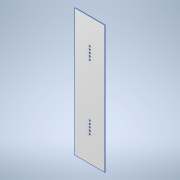
# Autodesk Inventor part: 7001_Aluminum_Chasis_Coil_Assembly_Separator_Tx_Filter_MPSv2_v1
Saved by Autodesk Inventor 2021 (Build 250183000, 183)
## iProperties
Created: 2020-11-18
Part Number: 7001_Aluminum_Chasis_Coil_Assembly_Separator_Tx_Filter_MPSv2_v1
Material: Aluminum 6061
Document SubType Name: Modeling
Designer: Admin
Density: 2.7 g/cm^3
Appearance: Aluminum - Flat
Author: Admin
Autodesk Inventor part; units mm, degrees
ref_plane "YZ Plane" through (0, 0, 0) normal (1, 0, 0) x (0, 1, 0)
ref_plane "XZ Plane" through (0, 0, 0) normal (0, 1, 0) x (-1, 0, 0)
ref_plane "XY Plane" through (0, 0, 0) normal (0, 0, 1) x (1, 0, 0)
sketch "Sketch1" plane through (0, 0, 0) normal (0, 0, 1) x (1, 0, 0)
  line L0 (0, 0) -> (101.5, 0)
  line L1 (101.5, 0) -> (101.5, -430)
  line L2 (101.5, -430) -> (0, -430)
  line L3 (0, -430) -> (0, 0)
  dimension "d0" = 101.5
  dimension "d1" = 430
  constraints: 8 end point, 2 parallel, 1 horizontal, 1 perpendicular
  measures "d0" distance of L1.end L2.end
  measures "d1" distance of L0.end L1.end
extrude "Extrusion1" add sketch "Sketch1" along normal blind 1.8
sketch "Sketch2" plane through (0, 0, 1.8) normal (0, 0, 1) x (1, 0, 0)
  line L0 (0, 0) -> (0, -430) projected
  line L1 (101.5, -430) -> (101.5, 0) projected
  line L2 (0, 0) -> (101.5, 0)
  line L3 (101.5, 0) -> (101.5, -10)
  line L4 (101.5, -10) -> (0, -10)
  line L5 (0, -10) -> (0, 0)
  line L6 (50.75, -10) -> (140.75, -10)
  line L7 (140.75, -10) -> (140.75, -106.4042)
  line L8 (140.75, -106.4042) -> (50.75, -106.4042)
  line L9 (50.75, -106.4042) -> (50.75, -10)
  circle A0 centre (50.75, -106.4042) radius 2.5
  line L10 (50.75, -106.4042) -> (50.75, -126.4042)
  circle A1 centre (50.75, -126.4042) radius 2.5
  line L11 (50.75, -106.4042) -> (50.75, -86.4042)
  circle A2 centre (50.75, -86.4042) radius 2.5
  circle A3 centre (50.75, -96.4042) radius 2.5
  circle A4 centre (50.75, -116.4042) radius 2.5
  line L12 (101.5, 0) -> (0, 0) projected
  line L13 (0, -430) -> (101.5, -430) projected
  line L14 (0, 0) -> (101.5, -430)
  line L15 (101.5, -430) -> (50.75, -215)
  line L16 (50.75, -215) -> (87.135, -215)
  circle A5 centre (50.75, -323.5958) radius 2.5
  line L17 (50.75, -323.5958) -> (50.75, -303.5958)
  circle A6 centre (50.75, -303.5958) radius 2.5
  line L18 (50.75, -323.5958) -> (50.75, -343.5958)
  circle A7 centre (50.75, -343.5958) radius 2.5
  circle A8 centre (50.75, -333.5958) radius 2.5
  circle A9 centre (50.75, -313.5958) radius 2.5
  dimension "d4" = 10
  dimension "d5" = 90
  dimension "d6" = 5
  dimension "d7" = 20
  dimension "d8" = 20
  dimension "d9" = 5
  dimension "d10" = 5
  dimension "d11" = 5
  constraints: 30 end point, 10 centre point, 8 symmetric about line, 6 coincident, 4 midpoint, 4 parallel, 3 horizontal, 2 perpendicular, 2 point on line, 1 vertical, 5 other
  measures "d4" distance of L2.end L3.end
  measures "d5" distance of L7.end L8.end
  measures "d6" diameter of A0
  measures "d7" distance of L10.start L10.end
  measures "d8" distance of L10.start L11.end
  measures "d9" diameter of A2
  measures "d10" diameter of A3
  measures "d11" diameter of A4
extrude "Extrusion2" cut sketch "Sketch2" against normal blind 10 contours A2 L9 | L9 A2 | A0 L10 L8 | L8 L9 A0 | L10 A0 L9 | A3 L9 | L9 A3 | A4 L10 | L10 A4 | A1 | A5 L18 L17 | L17 L18 A5 | A9 L17 | L17 A9 | A6 | A8 L18 | L18 A8 | A7
body "Solid1"
